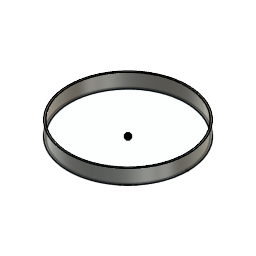
TPU_Belt (Autodesk Fusion 360 design; units mm, degrees)
Autodesk Fusion 360 part; units mm, degrees
sketch "Sketch1" plane through (0, 0, 0) normal (0, 0, 1) x (1, 0, 0)
  circle A0 centre (0, 0) radius 32.1493
  circle A1 centre (0, 0) radius 33.0493
  dimension "d1" = 64.2987
  dimension "d4" = 66.0987
  constraint coincident A0.centre A1.centre
  measures "d1" diameter of A0
  measures "d4" diameter of A1
extrude "Extrude1" add sketch "Sketch1" along normal blind 8
equation "d1 = inner_diameter"
equation "inner_circumference = 202 mm"
equation "inner_diameter = inner_circumference / 3.14159"
equation "d4 = inner_diameter + belt_thickness"
equation "d5 = belt_width"
equation "belt_width = 8 mm"
equation "belt_thickness = 1.8 mm"
named bodies: "TPU_Belt"
